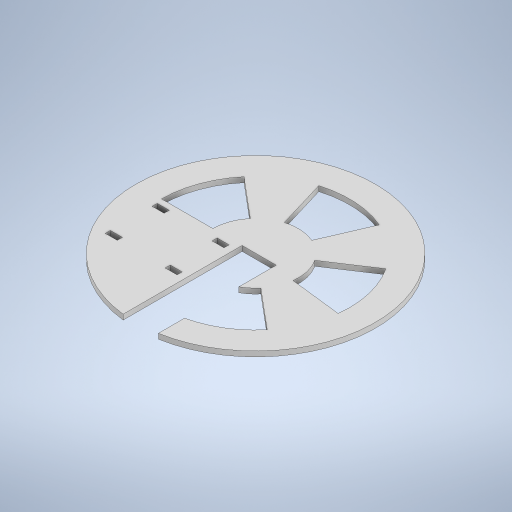
# Autodesk Inventor part: 轉盤
Saved by Autodesk Inventor 2024 (Build 280153000, 153)
## iProperties
Created: 2024-03-31
Part Number: 轉盤
Material: 一般
Document SubType Name: Modeling
Designer: USER
Density: 1 g/cm^3
Appearance: 預設
Author: USER
Autodesk Inventor part; units mm, degrees
ref_plane "YZ Plane" through (0, 0, 0) normal (1, 0, 0) x (0, 1, 0)
ref_plane "XZ Plane" through (0, 0, 0) normal (0, 1, 0) x (-1, 0, 0)
ref_plane "XY Plane" through (0, 0, 0) normal (0, 0, 1) x (1, 0, 0)
sketch "草圖3" plane through (0, 0, 0) normal (0, 1, 0) x (-1, 0, 0)
  circle A0 centre (0, 0) radius 25
  circle A1 centre (0, 0) radius 70
  line L0 (5, 5) -> (61, 5)
  line L1 (61, 5) -> (61, 32.4)
  line L2 (61, 32.4) -> (5, 32.4)
  line L3 (5, 32.4) -> (5, 5)
  line L4 (19, 33.9) -> (12, 33.9)
  line L5 (12, 33.9) -> (12, 30.9)
  line L6 (12, 30.9) -> (19, 30.9)
  line L7 (19, 30.9) -> (19, 33.9)
  line L8 (54, 33.9) -> (47, 33.9)
  line L9 (47, 33.9) -> (47, 30.9)
  line L10 (47, 30.9) -> (54, 30.9)
  line L11 (54, 30.9) -> (54, 33.9)
  line L12 (61, 18.7) -> (5, 18.7)
  line L13 (19, 3.5) -> (12, 3.5)
  line L14 (12, 3.5) -> (12, 6.5)
  line L15 (12, 6.5) -> (19, 6.5)
  line L16 (19, 6.5) -> (19, 3.5)
  line L17 (54, 3.5) -> (47, 3.5)
  line L18 (47, 3.5) -> (47, 6.5)
  line L19 (47, 6.5) -> (54, 6.5)
  line L20 (54, 6.5) -> (54, 3.5)
  line L21 (0, 0) -> (55, 0)
  line L22 (19.1511, -16.0697) -> (42.1324, -35.3533)
  arc A2 (42.1324, -35.3533) -> (55, 0) centre (0, 0) ccw
  line L23 (0, 0) -> (15.7742, -52.6894)
  arc A3 (-21.7844, -50.5019) -> (15.7742, -52.6894) centre (0, 0) ccw
  line L24 (-9.902, -22.9554) -> (-21.7844, -50.5019)
  line L25 (0, 0) -> (-45.9518, -30.223)
  arc A4 (-54.6281, 6.3851) -> (-45.9518, -30.223) centre (0, 0) ccw
  line L26 (-24.831, 2.9023) -> (-54.6281, 6.3851)
  line L27 (0, 0) -> (-42.1324, 35.3533)
  arc A5 (-9.5506, 54.1644) -> (-42.1324, 35.3533) centre (0, 0) ccw
  line L28 (-4.3412, 24.6202) -> (-9.5506, 54.1644)
  line L29 (17.5, 0) -> (-21.7065, 0)
  line L30 (7.8968, 70) -> (-12.1032, 70)
  line L31 (-12.1032, 70) -> (-12.1032, 0)
  line L32 (-12.1032, 0) -> (7.8968, 0)
  line L33 (7.8968, 0) -> (7.8968, 70)
  point P0 (25, 0)
  point P1 (12, 32.4)
  point P2 (47, 32.4)
  point P3 (12, 5)
  point P4 (47, 5)
  point P5 (0, -70)
  point P6 (-20.8872, -13.7377)
  point P7 (-19.1511, 16.0697)
  point P8 (-4.3412, 24.6202)
  point P9 (25, 0)
  point P10 (-2.1032, 0)
  point P11 (7.1701, -23.9497)
  point P12 (-9.902, -22.9554)
  point P13 (-12.1032, 21.8749)
  point P14 (-12.1032, 33.2534)
  point P15 (-12.1032, 68.9457)
  point P16 (7.8968, 69.5532)
  point P17 (7.8968, 23.7201)
  point P18 (-12.1032, 53.6518)
  point P19 (0, 70)
  point P20 (-12.1032, 10.1558)
  dimension "d19" = 140
  dimension "d30" = 56
  dimension "d31" = 27.4
  dimension "d32" = 5
  dimension "d34" = 3
  dimension "d35" = 7
  dimension "d36" = 3
  dimension "d37" = 7
  dimension "d38" = 7
  dimension "d39" = 7
  dimension "d48" = 50
  dimension "d54" = 36
  dimension "d55" = 55
  dimension "d56" = 40
  dimension "d57" = 0
  dimension "d60" = 220
  dimension "d62" = 20
  dimension "d63" = 70
  dimension "d64" = 53.1032
  dimension "d65" = 30.9
  dimension "d66" = 36
  dimension "d67" = 30.9
  dimension "d68" = 43.5
  dimension "d69" = 61
  dimension "d70" = 30.9
  dimension "d71" = 61
  dimension "d72" = 30.9
  dimension "d73" = 100.9
  dimension "d74" = 69.5505
  dimension "d75" = 7.4077
  dimension "d76" = 80.1511
  dimension "d77" = 46.9697
  dimension "d78" = 82.6506
  dimension "d79" = 18.4
  dimension "d80" = 86
  dimension "d81" = 30.9
  constraints: 68 end point, 10 point on circle, 10 symmetric about line, 8 parallel, 7 coincident, 6 centre point, 6 midpoint, 5 horizontal, 4 horizontal alignment, 4 perpendicular, 1 collinear, 1 vertical alignment, 25 other
  measures "d19" diameter of A1
  measures "d30" distance of L1.end L2.end
  measures "d31" distance of L0.end L1.end
  measures "d32" horizontal distance of point (0, 0) L0.start
  measures "d34" distance of L10.end L8.start
  measures "d35" distance of L9.end L10.end
  measures "d36" distance of L6.end L4.start
  measures "d37" distance of L5.end L6.end
  measures "d38" horizontal distance of L2.end L5.end
  measures "d39" horizontal distance of L1.end L8.start
  measures "d48" diameter of A0
  measures "d54" distance from line of A0.start L1
  measures "d55" distance of L21.start L21.end
  measures "d56" angle of L21 L22
  measures "d57" distance from line of point (0, 0) L22
  measures "d62" distance of L31.end L32.end
  measures "d63" distance of L30.end L31.end
  measures "d64" distance between parallel lines of L33 L1
  measures "d65" distance between parallel lines of L10 L21
  measures "d66" distance from line of point (25, 0) L1
  measures "d67" distance from line of point (25, 0) L10
  measures "d68" distance from line of L29.start L1
  measures "d69" distance from line of point (0, 0) L1
  measures "d70" distance from line of point (0, 0) L10
  measures "d71" distance from line of point (0, 0) L1
  measures "d72" distance from line of point (0, 0) L10
  measures "d73" distance from line of point (0, -70) L10
extrude "擠出2" add sketch "草圖3" against normal blind 3 contours A0 L23 L21 | L22 A2 L21 A0 L0 L18 L17 L20 L1 L2 L11 L8 L9 L7 L4 L5 L33 A1 L31 A5 L27 L26 A4 L25 L24 A3 L23 | L21 L33 L0 L14 L13 L16 A0 | A0 L25 L23 | L0 L16 L15 L14 L33 L12 A0 | A0 L12 L1 L0 L20 L19 L18 | L25 A0 L27 L31 L29 | L12 L33 A0 | A0 L33 L2 L5 L6 L7 L9 L10 L11 L1 L12 | L27 A0 L31
